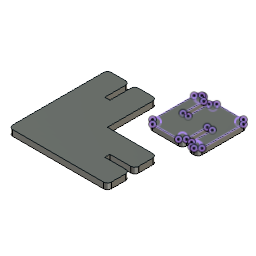
Construction kit 1 (Autodesk Fusion 360 design; units mm, degrees)
part number: 2026-02-07-16-20-51-833
Autodesk Fusion 360 part; units mm, degrees
sketch "Sketch1" plane through (0, 0, 0) normal (0, 0, 1) x (1, 0, 0)
sketch "Sketch2" plane through (0, 0, 0) normal (0, 0, 1) x (1, 0, 0)
  line L0 (0, 50) -> (0, 0)
  line L1 (0, 0) -> (50, 0)
  line L2 (50, 0) -> (50, 25)
  line L3 (50, 25) -> (25, 25)
  line L4 (25, 25) -> (25, 50)
  line L5 (25, 50) -> (0, 50)
  line L6 (12.5, 50) -> (12.5, 0) construction
  line L7 (0, 12.5) -> (50, 12.5) construction
  line L8 (11.2, 50) -> (11.2, 37.5)
  line L9 (11.2, 37.5) -> (13.8, 37.5)
  line L10 (13.8, 37.5) -> (13.8, 50)
  line L11 (50, 13.8) -> (37.5, 13.8)
  line L12 (37.5, 13.8) -> (37.5, 11.2)
  line L13 (37.5, 11.2) -> (50, 11.2)
  line L14 (33.0874, 37.7114) -> (33.0874, 62.7114)
  line L15 (33.0874, 62.7114) -> (58.0874, 62.7114)
  line L16 (58.0874, 62.7114) -> (58.0874, 37.7114)
  line L17 (58.0874, 37.7114) -> (33.0874, 37.7114)
  line L18 (45.5874, 62.7114) -> (45.5874, 37.7114) construction
  line L19 (39.3374, 62.7114) -> (39.3374, 38) construction
  line L20 (51.8374, 62.7114) -> (51.8374, 37.7114) construction
  line L21 (37.9943, 62.7114) -> (37.9943, 50.2114)
  line L22 (37.9943, 50.2114) -> (40.5943, 50.2114)
  line L23 (40.5943, 50.2114) -> (40.5943, 62.7114)
  line L24 (50.2359, 37.7114) -> (50.2359, 50.2114)
  line L25 (50.2359, 50.2114) -> (52.8359, 50.2114)
  line L26 (52.8359, 50.2114) -> (52.8359, 37.7114)
  dimension "d5" = 50
  dimension "d6" = 2.6
  dimension "d7" = 2.6
  dimension "d8" = 12.5
  dimension "d9" = 12.5
  dimension "d18" = 25
  dimension "d19" = 25
  dimension "d20" = 2.6
  dimension "d21" = 2.6
  dimension "d22" = 12.5
  dimension "d23" = 12.5
  constraint coincident L0.end L1.start
  constraint vertical L0
  constraint perpendicular L2 L3
  constraint parallel L0 L4
  constraint perpendicular L0 L5
  constraint vertical L2
  constraint perpendicular L0 L1
  constraint equal L4 L5
  constraint equal L3 L4
  constraint equal L0 L1
  constraint midpoint L5 L6.start
  constraint coincident L1 L6.end
  constraint perpendicular L1 L6
  constraint coincident L0 L7.start
  constraint perpendicular L0 L7
  constraint coincident L2 L7.end
  constraint coincident L5 L8.start
  constraint perpendicular L5 L8
  constraint perpendicular L0 L9
  constraint coincident L5 L10.end
  constraint perpendicular L5 L10
  constraint coincident L2 L11.start
  constraint perpendicular L2 L11
  constraint perpendicular L11 L12
  constraint coincident L2 L13.end
  constraint perpendicular L2 L13
  constraint symmetric L7 L11 L13
  constraint perpendicular L14 L15
  constraint perpendicular L15 L16
  constraint horizontal L17
  constraint perpendicular L14 L17
  constraint coincident L15 L18.start
  constraint perpendicular L15 L18
  constraint coincident L17 L18.end
  constraint symmetric L14 L16 L18
  constraint coincident L15 L19.start
  constraint perpendicular L15 L19
  constraint coincident L15 L20.start
  constraint perpendicular L15 L20
  constraint coincident L17 L20.end
  constraint coincident L15 L21.start
  constraint perpendicular L15 L21
  constraint perpendicular L19 L22
  constraint coincident L15 L23.end
  constraint perpendicular L15 L23
  constraint coincident L17 L24.start
  constraint perpendicular L17 L24
  constraint perpendicular L20 L25
  constraint coincident L17 L26.end
  constraint perpendicular L17 L26
  measures "d5" distance of L1 L5
  measures "d6" distance of L11 L13
  measures "d7" distance of L8 L10
  measures "d8" distance of L5 L9
  measures "d9" distance of L2 L12
  measures "d18" distance of L14 L16
  measures "d19" distance of L15 L17
  measures "d20" distance of L21 L23
  measures "d21" distance of L24 L26
  measures "d22" distance of L15 L22
  measures "d23" distance of L17 L25
extrude "Extrude1" add sketch "Sketch2" along normal blind 3 contours L0 L1 L2 L3 L4 L5 L8 L9 L10 L11 L12 L13 makes body 1
fillet "Fillet1" radius 2 4 edges at (13.8, 50, 1.5) (11.2, 50, 1.5) (0, 50, 1.5) (25, 50, 1.5) on bodies 1
fillet "Fillet2" radius 2 4 edges at (50, 25, 1.5) (50, 13.8, 1.5) (50, 11.2, 1.5) (50, 0, 1.5) on bodies 1
fillet "Fillet3" radius 2 1 edges at (0, 0, 1.5) on bodies 1
extrude "Extrude2" add sketch "Sketch2" along normal blind 3 separate body contours L14 L15 L16 L17 L21 L22 L23 L24 L25 L26 makes body 2
fillet "Fillet4" radius 2 8 edges at (58.0874, 37.7114, 1.5) (52.8359, 37.7114, 1.5) (50.2359, 37.7114, 1.5) (33.0874, 37.7114, 1.5) (33.0874, 62.7114, 1.5) (37.9943, 62.7114, 1.5) (40.5943, 62.7114, 1.5) (58.0874, 62.7114, 1.5) on bodies 2
sketch "Sketch5" plane through (0, 0, 3) normal (0, 0, 1) x (-1, 0, 0)
  arc A0 (0, -2) -> (-2, 0) centre (-2, -2) ccw
  line L0 (-2, 0) -> (-48, 0)
  arc A1 (-48, 0) -> (-50, -2) centre (-48, -2) ccw
  line L1 (-50, -2) -> (-50, -9.2)
  arc A2 (-50, -9.2) -> (-48, -11.2) centre (-48, -9.2) ccw
  line L2 (-48, -11.2) -> (-37.5, -11.2)
  line L3 (-37.5, -11.2) -> (-37.5, -13.8)
  line L4 (-37.5, -13.8) -> (-48, -13.8)
  arc A3 (-48, -13.8) -> (-50, -15.8) centre (-48, -15.8) ccw
  line L5 (-50, -15.8) -> (-50, -23)
  arc A4 (-50, -23) -> (-48, -25) centre (-48, -23) ccw
  line L6 (-48, -25) -> (-25, -25)
  line L7 (-25, -25) -> (-25, -48)
  arc A5 (-25, -48) -> (-23, -50) centre (-23, -48) ccw
  line L8 (-23, -50) -> (-15.8, -50)
  arc A6 (-15.8, -50) -> (-13.8, -48) centre (-15.8, -48) ccw
  line L9 (-13.8, -48) -> (-13.8, -37.5)
  line L10 (-13.8, -37.5) -> (-11.2, -37.5)
  line L11 (-11.2, -37.5) -> (-11.2, -48)
  arc A7 (-11.2, -48) -> (-9.2, -50) centre (-9.2, -48) ccw
  line L12 (-9.2, -50) -> (-2, -50)
  arc A8 (-2, -50) -> (0, -48) centre (-2, -48) ccw
  line L13 (0, -48) -> (0, -2)
sketch "Sketch6" plane through (0, 0, 3) normal (0, 0, 1) x (-1, 0, 0)
  arc A0 (-58.0874, -60.7114) -> (-56.0874, -62.7114) centre (-56.0874, -60.7114) ccw
  line L0 (-56.0874, -62.7114) -> (-42.5943, -62.7114)
  arc A1 (-42.5943, -62.7114) -> (-40.5943, -60.7114) centre (-42.5943, -60.7114) ccw
  line L1 (-40.5943, -60.7114) -> (-40.5943, -50.2114)
  line L2 (-40.5943, -50.2114) -> (-37.9943, -50.2114)
  line L3 (-37.9943, -50.2114) -> (-37.9943, -60.7114)
  arc A2 (-37.9943, -60.7114) -> (-35.9943, -62.7114) centre (-35.9943, -60.7114) ccw
  arc A3 (-35.0874, -62.7114) -> (-33.0874, -60.7114) centre (-35.0874, -60.7114) ccw
  line L4 (-33.0874, -60.7114) -> (-33.0874, -39.7114)
  arc A4 (-33.0874, -39.7114) -> (-35.0874, -37.7114) centre (-35.0874, -39.7114) ccw
  line L5 (-35.0874, -37.7114) -> (-48.2359, -37.7114)
  arc A5 (-48.2359, -37.7114) -> (-50.2359, -39.7114) centre (-48.2359, -39.7114) ccw
  line L6 (-50.2359, -39.7114) -> (-50.2359, -50.2114)
  line L7 (-50.2359, -50.2114) -> (-52.8359, -50.2114)
  line L8 (-52.8359, -50.2114) -> (-52.8359, -39.7114)
  arc A6 (-52.8359, -39.7114) -> (-54.8359, -37.7114) centre (-54.8359, -39.7114) ccw
  arc A7 (-56.0874, -37.7114) -> (-58.0874, -39.7114) centre (-56.0874, -39.7114) ccw
  line L9 (-58.0874, -39.7114) -> (-58.0874, -60.7114)
  line L10 (-35.9943, -62.7114) -> (-35.0874, -62.7114)
  line L11 (-54.8359, -37.7114) -> (-56.0874, -37.7114)
sketch "Sketch7" plane through (0, 0, 3) normal (0, 0, 1) x (-1, 0, 0)
  arc A0 (0, -2) -> (-2, 0) centre (-2, -2) ccw
  line L0 (-2, 0) -> (-48, 0)
  arc A1 (-48, 0) -> (-50, -2) centre (-48, -2) ccw
  line L1 (-50, -2) -> (-50, -9.2)
  arc A2 (-50, -9.2) -> (-48, -11.2) centre (-48, -9.2) ccw
  line L2 (-48, -11.2) -> (-37.5, -11.2)
  line L3 (-37.5, -11.2) -> (-37.5, -13.8)
  line L4 (-37.5, -13.8) -> (-48, -13.8)
  arc A3 (-48, -13.8) -> (-50, -15.8) centre (-48, -15.8) ccw
  line L5 (-50, -15.8) -> (-50, -23)
  arc A4 (-50, -23) -> (-48, -25) centre (-48, -23) ccw
  line L6 (-48, -25) -> (-25, -25)
  line L7 (-25, -25) -> (-25, -48)
  arc A5 (-25, -48) -> (-23, -50) centre (-23, -48) ccw
  line L8 (-23, -50) -> (-15.8, -50)
  arc A6 (-15.8, -50) -> (-13.8, -48) centre (-15.8, -48) ccw
  line L9 (-13.8, -48) -> (-13.8, -37.5)
  line L10 (-13.8, -37.5) -> (-11.2, -37.5)
  line L11 (-11.2, -37.5) -> (-11.2, -48)
  arc A7 (-11.2, -48) -> (-9.2, -50) centre (-9.2, -48) ccw
  line L12 (-9.2, -50) -> (-2, -50)
  arc A8 (-2, -50) -> (0, -48) centre (-2, -48) ccw
  line L13 (0, -48) -> (0, -2)
  arc A9 (-58.0874, -60.7114) -> (-56.0874, -62.7114) centre (-56.0874, -60.7114) ccw
  line L14 (-56.0874, -62.7114) -> (-42.5943, -62.7114)
  arc A10 (-42.5943, -62.7114) -> (-40.5943, -60.7114) centre (-42.5943, -60.7114) ccw
  line L15 (-40.5943, -60.7114) -> (-40.5943, -50.2114)
  line L16 (-40.5943, -50.2114) -> (-37.9943, -50.2114)
  line L17 (-37.9943, -50.2114) -> (-37.9943, -60.7114)
  arc A11 (-37.9943, -60.7114) -> (-35.9943, -62.7114) centre (-35.9943, -60.7114) ccw
  line L18 (-35.9943, -62.7114) -> (-35.0874, -62.7114)
  arc A12 (-35.0874, -62.7114) -> (-33.0874, -60.7114) centre (-35.0874, -60.7114) ccw
  line L19 (-33.0874, -60.7114) -> (-33.0874, -39.7114)
  arc A13 (-33.0874, -39.7114) -> (-35.0874, -37.7114) centre (-35.0874, -39.7114) ccw
  line L20 (-35.0874, -37.7114) -> (-48.2359, -37.7114)
  arc A14 (-48.2359, -37.7114) -> (-50.2359, -39.7114) centre (-48.2359, -39.7114) ccw
  line L21 (-50.2359, -39.7114) -> (-50.2359, -50.2114)
  line L22 (-50.2359, -50.2114) -> (-52.8359, -50.2114)
  line L23 (-52.8359, -50.2114) -> (-52.8359, -39.7114)
  arc A15 (-52.8359, -39.7114) -> (-54.8359, -37.7114) centre (-54.8359, -39.7114) ccw
  line L24 (-54.8359, -37.7114) -> (-56.0874, -37.7114)
  arc A16 (-56.0874, -37.7114) -> (-58.0874, -39.7114) centre (-56.0874, -39.7114) ccw
  line L25 (-58.0874, -39.7114) -> (-58.0874, -60.7114)
equation "Kerf = 0.3 mm"
equation "Side = 50 mm"
equation "Width = 3 mm"
equation "d5 = Side"
equation "d6 = d7"
equation "d7 = Width - Kerf - Compression"
equation "d8 = Side / 4"
equation "d9 = Side / 4"
equation "d10 = Width"
equation "d13 = Fillet"
equation "d15 = Fillet"
equation "d17 = Fillet"
equation "d18 = Side / 2"
equation "d19 = Side / 2"
equation "d20 = d7"
equation "d21 = d7"
equation "d22 = Side / 4"
equation "d23 = Side / 4"
equation "d24 = Width"
equation "d27 = Fillet"
equation "Fillet = 2 mm"
equation "Compression = 0.1 mm"
